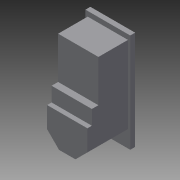
# Autodesk Inventor part: PowerSocket
Saved by Autodesk Inventor 2014 SP1 (Build 180222100, 222)
## iProperties
Created: 2014-01-01
Part Number: PowerSocket
Material: Generic
Document SubType Name: Modeling
Designer: Jack
Density: 1 g/cm^3
Appearance: Default
Author: Jack
Autodesk Inventor part; units mm, degrees
ref_plane "YZ Plane" through (0, 0, 0) normal (1, 0, 0) x (0, 1, 0)
ref_plane "XZ Plane" through (0, 0, 0) normal (0, 1, 0) x (-1, 0, 0)
ref_plane "XY Plane" through (0, 0, 0) normal (0, 0, 1) x (1, 0, 0)
sketch "Sketch1" plane through (0, 0, 0) normal (0, 1, 0) x (-1, 0, 0)
  line L0 (0, 0) -> (30, 0)
  line L1 (30, 0) -> (30, 66.3)
  line L2 (30, 66.3) -> (0, 66.3)
  line L3 (0, 66.3) -> (0, 0)
  dimension "d0" = 30
  dimension "d1" = 66.3
  constraints: 8 end point, 2 parallel, 1 horizontal, 1 perpendicular
  measures "d0" distance of L0.start L0.end
  measures "d1" distance of L0.end L1.end
extrude "Extrusion1" add sketch "Sketch1" along normal blind 3.3
sketch "Sketch2" plane through (0, 0, 0) normal (0, -1, 0) x (1, 0, 0)
  line L0 (0, 0) -> (-30, 0) projected
  line L1 (0, 66.3) -> (0, 0) projected
  line L2 (-30, 66.3) -> (0, 66.3) projected
  line L3 (-30, 0) -> (-30, 66.3) projected
  line L4 (-28.5, 63) -> (-1.5, 63)
  line L5 (-28.5, 63) -> (-28.5, 11.3)
  line L6 (-20.5, 3.3) -> (-9.5, 3.3)
  line L7 (-1.5, 11.3) -> (-1.5, 63)
  line L8 (-9.5, 3.3) -> (-1.5, 11.3)
  line L9 (-28.5, 11.3) -> (-20.5, 3.3)
  point P0 (-28.5, 3.3)
  point P1 (-1.5, 3.3)
  dimension "d4" = 3.3
  dimension "d5" = 27
  dimension "d6" = 1.5
  dimension "d8" = 3.3
  dimension "d9" = 8
  dimension "d10" = 8
  dimension "d11" = 8
  dimension "d12" = 8
  constraints: 12 end point, 4 point on line, 3 perpendicular, 1 parallel
  measures "d4" distance between parallel lines of L2 L4
  measures "d5" distance of L4.start L4.end
  measures "d6" distance from line of L3 L4.start
  measures "d8" distance between parallel lines of L0 L6
  measures "d9" distance of L6.end point (-1.5, 3.3)
  measures "d10" distance of L7.start point (-1.5, 3.3)
  measures "d11" distance of L5.end point (-28.5, 3.3)
  measures "d12" distance of L6.start point (-28.5, 3.3)
extrude "Extrusion2" add sketch "Sketch2" along normal blind 19.8 contours L4 L7 L8 L6 L9 L5
sketch "Sketch3" plane through (0, -19.8, 0) normal (0, -1, 0) x (1, 0, 0)
  line L0 (-1.5, 63) -> (-28.5, 63) projected
  line L1 (-28.5, 63) -> (-28.5, 11.3) projected
  line L2 (-28.5, 11.3) -> (-20.5, 3.3) projected
  line L3 (-20.5, 3.3) -> (-9.5, 3.3) projected
  line L4 (-9.5, 3.3) -> (-1.5, 11.3) projected
  line L5 (-1.5, 11.3) -> (-1.5, 63) projected
  line L6 (-28.5, 35) -> (-1.5, 35)
  point P0 (0, 0)
  dimension "d15" = 28
  constraints: 2 end point, 2 point on line, 1 perpendicular
  measures "d15" distance between parallel lines of L0 L6
extrude "Extrusion3" add sketch "Sketch3" along normal blind 4.4 contours L5 L4 L3 L2 L1 L6
sketch "Sketch4" plane through (0, -24.2, 0) normal (0, -1, 0) x (1, 0, 0)
  line L0 (-28.5, 11.3) -> (-20.5, 3.3) projected
  line L1 (-20.5, 3.3) -> (-9.5, 3.3) projected
  line L2 (-9.5, 3.3) -> (-1.5, 11.3) projected
  line L3 (-1.5, 11.3) -> (-1.5, 35) projected
  line L4 (-1.5, 35) -> (-28.5, 35) projected
  line L5 (-28.5, 35) -> (-28.5, 11.3) projected
  line L6 (-28.5, 25.3) -> (-1.5, 25.3)
  point P0 (0, 0)
  dimension "d18" = 9.7
  constraints: 2 end point, 2 point on line, 1 perpendicular
  measures "d18" distance between parallel lines of L4 L6
extrude "Extrusion4" add sketch "Sketch4" along normal blind 3 contours L5 L6 L3 L2 L1 L0
sketch "Sketch5" plane through (0, 3.3, 0) normal (0, 1, 0) x (1, 0, 0)
  line L0 (0, 0) -> (-30, 0) projected
  line L1 (-30, 0) -> (-30, -66.3) projected
  line L2 (0, -66.3) -> (0, 0) projected
  line L3 (-3, -21.3) -> (-3, -10)
  line L4 (-8, -5) -> (-22, -5)
  line L5 (-27, -10) -> (-27, -21.3)
  line L6 (-27, -21.3) -> (-3, -21.3)
  line L7 (-3, -10) -> (-8, -5)
  line L8 (-27, -10) -> (-22, -5)
  point P0 (-3, -5)
  point P1 (-27, -5)
  dimension "d21" = 16.3
  dimension "d22" = 24
  dimension "d24" = 3
  dimension "d25" = 5
  dimension "d26" = 5
  dimension "d27" = 5
  dimension "d28" = 5
  dimension "d29" = 5
  constraints: 12 end point, 4 point on line, 2 parallel, 1 horizontal, 1 perpendicular
  measures "d21" distance of L3.start point (-3, -5)
  measures "d22" distance of point (-3, -5) point (-27, -5)
  measures "d24" distance between parallel lines of L2 L3
  measures "d25" distance between parallel lines of L0 L4
  measures "d26" distance of L3.end point (-3, -5)
  measures "d27" distance of L4.start point (-3, -5)
  measures "d28" distance of L5.start point (-27, -5)
  measures "d29" distance of L4.end point (-27, -5)
extrude "Extrusion5" cut sketch "Sketch5" against normal blind 19
sketch "Sketch6" plane through (0, -15.7, 0) normal (0, 1, 0) x (1, 0, 0)
  line L0 (-22, -5) -> (-8, -5) projected
  line L1 (-27, -21.3) -> (-27, -10) projected
  line L2 (-3, -21.3) -> (-27, -21.3) projected
  line L3 (-22.75, -13.3) -> (-22.75, -17.3)
  line L4 (-22.75, -17.3) -> (-20.75, -17.3)
  line L5 (-20.75, -17.3) -> (-20.75, -13.3)
  line L6 (-20.75, -13.3) -> (-22.75, -13.3)
  line L7 (-9.25, -13.3) -> (-9.25, -17.3)
  line L8 (-9.25, -17.3) -> (-7.25, -17.3)
  line L9 (-7.25, -17.3) -> (-7.25, -13.3)
  line L10 (-7.25, -13.3) -> (-9.25, -13.3)
  line L11 (-8.25, -13.3) -> (-8.25, -17.3) construction
  line L12 (-21.75, -13.3) -> (-21.75, -17.3) construction
  line L13 (-16, -9) -> (-16, -13)
  line L14 (-16, -13) -> (-14, -13)
  line L15 (-14, -13) -> (-14, -9)
  line L16 (-14, -9) -> (-16, -9)
  point P0 (0, 0)
  dimension "d32" = 2
  dimension "d33" = 2
  dimension "d34" = 13.5
  dimension "d35" = 4
  dimension "d36" = 4
  dimension "d37" = 5.25
  dimension "d38" = 4
  dimension "d39" = 4
  dimension "d40" = 2
  dimension "d41" = 4
  dimension "d42" = 4.75
  constraints: 28 end point, 8 perpendicular, 4 midpoint, 4 parallel, 1 horizontal alignment
  measures "d32" distance between parallel lines of L5 L3
  measures "d33" distance of L7.end L8.end
  measures "d34" distance between parallel lines of L11 L12
  measures "d35" distance between parallel lines of L4 L6
  measures "d36" distance between parallel lines of L8 L10
  measures "d37" distance between parallel lines of L1 L12
  measures "d38" distance between parallel lines of L2 L4
  measures "d39" distance of L13.start L13.end
  measures "d40" distance of L13.end L14.end
  measures "d41" distance between parallel lines of L0 L16
  measures "d42" distance between parallel lines of L7 L15
extrude "Extrusion6" add sketch "Sketch6" along normal blind 15
equation "\"d10\" = d9"
equation "\"d12\" = d11"
equation "\"d27\" = d26"
equation "\"d29\" = d28"
body "Solid1"
